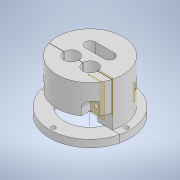
# Autodesk Inventor part: big_actuator_holder
Saved by Autodesk Inventor 2021 (Build 250183000, 183)
## iProperties
Created: 2020-10-24
Part Number: big_actuator_holder
Material: Generic
Document SubType Name: Modeling
Designer: bober
Density: 1 g/cm^3
Appearance: Default
Author: bober
Autodesk Inventor part; units mm, degrees
ref_plane "YZ Plane" through (0, 0, 0) normal (1, 0, 0) x (0, 1, 0)
ref_plane "XZ Plane" through (0, 0, 0) normal (0, 1, 0) x (-1, 0, 0)
ref_plane "XY Plane" through (0, 0, 0) normal (0, 0, 1) x (1, 0, 0)
sketch "Sketch1" plane through (0, 0, 0) normal (0, 1, 0) x (-1, 0, 0)
  line L0 (-6.7037, 6.5) -> (6.2963, 6.5)
  line L1 (6.2963, 6.5) -> (6.2963, -6.5)
  line L2 (6.2963, -6.5) -> (-6.7037, -6.5)
  line L3 (-6.7037, -6.5) -> (-6.7037, 6.5)
  line L4 (-6.7037, 6.5) -> (6.2963, -6.5) construction
  line L5 (6.2963, 6.5) -> (-6.7037, -6.5) construction
  circle A0 centre (6.2963, 6.5) radius 5.045
  circle A1 centre (-6.7037, 6.5) radius 5.045
  line L6 (6.2963, -6.5) -> (-6.7037, -6.5) construction
  line L7 (6.2963, -3) -> (-6.7037, -3)
  line L8 (-6.7037, -10) -> (6.2963, -10)
  arc A2 (6.2963, -10) -> (6.2963, -3) centre (6.2963, -6.5) ccw
  arc A3 (-6.7037, -3) -> (-6.7037, -10) centre (-6.7037, -6.5) ccw
  circle A4 centre (0, 0) radius 22.5
  line L9 (-23.7037, 6.6) -> (36.2963, 6.6)
  line L10 (36.2963, 6.6) -> (36.2963, 6.4)
  line L11 (36.2963, 6.4) -> (-23.7037, 6.4)
  line L12 (-23.7037, 6.4) -> (-23.7037, 6.6)
  line L13 (-23.7037, 6.6) -> (36.2963, 6.4) construction
  line L14 (36.2963, 6.6) -> (-23.7037, 6.4) construction
  point P0 (-0.2037, 0)
  point P1 (-0.2037, -6.5)
  point P2 (11.3403, 6.6)
  point P3 (21.5102, 6.6)
  point P4 (-21.5102, 6.6)
  point P5 (-11.7478, 6.6)
  point P6 (-1.6597, 6.6)
  point P7 (1.2522, 6.6)
  point P8 (1.2522, 6.4)
  point P9 (-1.6597, 6.4)
  point P10 (-11.7478, 6.4)
  point P11 (-21.5706, 6.4)
  point P12 (21.5706, 6.4)
  point P13 (11.3403, 6.4)
  dimension "d0" = 13
  dimension "d1" = 13
  dimension "d2" = 10.09
  dimension "d3" = 10.09
  dimension "d4" = 7
  dimension "d5" = 45
  dimension "d6" = 60
  dimension "d7" = 0.2
  constraints: 32 end point, 5 centre point, 5 midpoint, 5 parallel, 4 point on circle, 4 tangent, 3 coincident, 3 horizontal, 2 perpendicular
  measures "d0" distance of L1.end L2.end
  measures "d1" distance of L0.end L1.end
  measures "d2" diameter of A0
  measures "d3" diameter of A1
  measures "d4" diameter of A3
  measures "d5" diameter of A4
  measures "d6" distance of L10.end L11.end
  measures "d7" distance of L9.end L10.end
extrude "Extrusion1" add sketch "Sketch1" along normal blind 20 contours A1 L9 A4 A0 | L11 A0 L1 L7 L3 A1 | L3 A3 L8 A2 L1 A0 L11 A4 A1
extrude "Extrusion2" add sketch "Sketch1" against normal blind 10 contours L11 A0 L1 L7 L3 A1 | L3 A3 L8 A2 L1 A0 L11 A4 A1
sketch "Sketch2" plane through (0, -10, 0) normal (0, -1, 0) x (1, 0, 0)
  circle A0 centre (0, 0) radius 17.5
  circle A1 centre (0, 0) radius 27.5
  dimension "d12" = 35
  dimension "d13" = 55
  constraints: 2 centre point, 2 coincident
  measures "d12" diameter of A0
  measures "d13" diameter of A1
extrude "Extrusion3" add sketch "Sketch2" along normal blind 5
sketch "Sketch3" plane through (0, -10, 0) normal (0, 1, 0) x (1, 0, 0)
  circle A0 centre (0, 25) radius 1.5
  point P0 (0, 0)
  dimension "d16" = 3
  constraints: 1 centre point
  measures "d16" diameter of A0
extrude "Extrusion4" cut sketch "Sketch3" against normal blind 5
pattern_circular "Circular Pattern1" count 4 over 360 about axis through (0, -10, 0) along (0, -1, 0) of "Extrusion4"
sketch "Sketch4" plane through (21.5102, 0, 6.6) normal (0, 0, -1) x (-1, 0, 0)
  circle A0 centre (4.8812, 5) radius 1.5
  point P0 (21.5102, 0)
  dimension "d22" = 3
  constraints: 1 centre point
  measures "d22" diameter of A0
extrude "Extrusion5" cut sketch "Sketch4" along normal blind 30 and the other way blind 15
ref_plane "Work Plane1" through (21.5102, 0, -8.4) normal (0, 0, -1) x (-1, 0, 0)
sketch "Sketch5" plane through (21.5102, 0, -8.4) normal (0, 0, -1) x (-1, 0, 0)
  circle A0 centre (4.8812, 5) radius 1.5 projected
  circle A1 centre (4.8812, 5) radius 2.75
  line L0 (2.1312, 6.5877) -> (4.8812, 8.1754)
  line L1 (4.8812, 8.1754) -> (7.6312, 6.5877)
  line L2 (7.6312, 6.5877) -> (7.6312, 3.4123)
  line L3 (7.6312, 3.4123) -> (4.8812, 1.8246)
  line L4 (4.8812, 1.8246) -> (2.1312, 3.4123)
  line L5 (2.1312, 3.4123) -> (2.1312, 6.5877)
  point P0 (21.5102, 0)
  point P1 (2.1312, 5)
  dimension "d28" = 5.5
  constraints: 12 end point, 2 coincident, 1 horizontal alignment, 1 midpoint, 15 other
extrude "Extrusion6" cut sketch "Sketch5" along normal blind 30 contours A0 | A1 | L2 L3 A1 | A1 L1 L2 | A1 L0 L1 | L3 L4 A1 | A1 L5 L0 | L4 L5 A1
mirror "Mirror1" about plane through (0, 0, 0) normal (1, 0, 0) of "Extrusion6", "Extrusion5"
ref_plane "Work Plane2" through (11.7478, 20, 6.4) normal (0, 0, 1) x (1, 0, 0)
ref_plane "Work Plane3" through (11.7478, 20, 12.4) normal (0, 0, 1) x (1, 0, 0)
sketch "Sketch8" plane through (11.7478, 20, 12.4) normal (0, 0, 1) x (1, 0, 0)
  circle A0 centre (4.8812, -15) radius 1.5 projected
  circle A1 centre (4.8812, -15) radius 4
  circle A2 centre (-28.3767, -15) radius 1.5 projected
  circle A3 centre (-28.3767, -15) radius 4
  line L0 (9.7625, -20) -> (0, -20) projected
  line L1 (8.8812, -15) -> (0.8812, -15)
  line L2 (0.8812, -15) -> (0.8812, -20)
  line L3 (0.8812, -20) -> (8.8812, -20)
  line L4 (8.8812, -20) -> (8.8812, -15)
  line L5 (9.7625, -20) -> (-33.258, -20) projected
  line L6 (-32.3767, -15) -> (-24.3767, -15)
  line L7 (-24.3767, -15) -> (-24.3767, -20)
  line L8 (-24.3767, -20) -> (-32.3767, -20)
  line L9 (-32.3767, -20) -> (-32.3767, -15)
  point P0 (-11.7478, -20)
  point P1 (0.8812, -15)
  point P2 (8.8812, -20)
  dimension "d35" = 8
  dimension "d36" = 8
  constraints: 16 end point, 4 parallel, 3 point on line, 2 coincident, 2 horizontal, 2 perpendicular, 6 other
extrude "Extrusion8" cut sketch "Sketch8" along normal blind 10 contours L1 A1 A0 | A0 L1 A1 | L4 L0 L2 A1 | L6 A3 A2 | A2 L6 A3 | L7 L5 L9 A3
split body "Split2" result two bodies by plane through (11.7478, 20, 6.4) normal (0, 0, 1) first body at (-5.0916, -10.5, 22.3331) (9.2654, 8.571, 19.9537)
body "Solid4"
body "Solid5"
